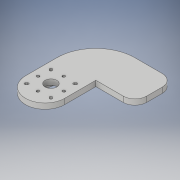
# Autodesk Inventor part: Motor Test Stand
Saved by Autodesk Inventor 2019 (Build 230136000, 136)
## iProperties
Created: 2019-09-23
Part Number: Motor Test Stand
Material: Generic
Document SubType Name: Modeling
Designer: isaac
Density: 1 g/cm^3
Appearance: Default
Author: isaac
Autodesk Inventor part; units mm, degrees
ref_plane "YZ Plane" through (0, 0, 0) normal (1, 0, 0) x (0, 1, 0)
ref_plane "XZ Plane" through (0, 0, 0) normal (0, 1, 0) x (-1, 0, 0)
ref_plane "XY Plane" through (0, 0, 0) normal (0, 0, 1) x (1, 0, 0)
sketch "Sketch1" plane through (0, 0, 0) normal (0, 1, 0) x (-1, 0, 0)
  line L0 (50, 65) -> (-50, 65)
  line L1 (-50, 65) -> (-50, -65)
  line L2 (-50, -65) -> (50, -65)
  line L3 (50, -65) -> (50, 65)
  line L4 (50, 65) -> (-50, -65) construction
  line L5 (-50, 65) -> (50, -65) construction
  point P0 (0, 0)
  dimension "d0" = 100
  dimension "d1" = 130
  constraints: 12 end point, 2 midpoint, 2 parallel, 1 horizontal, 1 perpendicular
  measures "d0" distance of L2.end L1.end
  measures "d1" distance of L1.end L0.end
extrude "Extrusion1" add sketch "Sketch1" along normal blind 7
sketch "Sketch2" plane through (0, 7, 0) normal (0, 1, 0) x (1, 0, 0)
  line L0 (-50, -65) -> (50, -65) projected
  line L1 (50, -65) -> (0, -65)
  line L2 (0, -65) -> (0, 0)
  line L3 (0, 0) -> (50, 0)
  line L4 (50, 0) -> (50, -65)
  constraints: 8 end point, 2 parallel, 1 horizontal, 1 perpendicular
extrude "Extrusion2" cut sketch "Sketch2" against normal up to next
fillet "Fillet1" radius 25 2 edges at (-50, 3.5, 65) (0, 3.5, 65)
sketch "Sketch5" plane through (0, 7, 0) normal (0, 1, 0) x (1, 0, 0)
  line L0 (-50, 65) -> (-50, -40) projected
  arc A0 (0, 50) -> (-50, 0) centre (0, 0) ccw
  line L1 (0, 50) -> (50, 50)
  line L2 (50, 0) -> (50, 65) projected
  line L3 (50, 50) -> (50, 65)
  line L4 (50, 65) -> (-50, 65) projected
  line L5 (50, 65) -> (-50, 65)
  line L6 (-50, 65) -> (-50, 0)
  constraints: 8 end point, 2 collinear, 2 point on circle, 1 centre point, 1 coincident, 1 horizontal, 1 perpendicular, 1 point on line, 1 tangent
extrude "Extrusion3" cut sketch "Sketch5" against normal up to next
fillet "Fillet2" radius 15 2 edges at (50, 3.5, 0) (50, 3.5, -50)
sketch "Sketch6" plane through (0, 7, 0) normal (0, 1, 0) x (1, 0, 0)
  arc A0 (0, 50) -> (-50, 0) centre (0, 0) ccw construction
  line L0 (-50, 0) -> (-25, -65) construction
  arc A1 (-50, -40) -> (0, -40) centre (-25, -40) ccw construction
  line L1 (0, -40) -> (0, 0) construction
  line L2 (0, 0) -> (-25, -65) construction
  line L3 (-25, -65) -> (-50, -65) construction
  line L4 (-50, 0) -> (-50, -40) construction
  line L5 (-50, -65) -> (-50, 0) construction
  line L6 (-25, -65) -> (0, -65) construction
  line L7 (0, -65) -> (0, 0) construction
  circle A2 centre (-25, -32.5) radius 22 construction
  line L8 (-47, -54.5) -> (-3, -54.5) construction
  line L9 (-3, -54.5) -> (-3, -10.5) construction
  line L10 (-3, -10.5) -> (-47, -10.5) construction
  line L11 (-47, -10.5) -> (-47, -54.5) construction
  line L12 (-47, -54.5) -> (-3, -10.5) construction
  line L13 (-3, -54.5) -> (-47, -10.5) construction
  line L14 (-41.0867, -48.5867) -> (-40.026, -47.526) construction
  line L15 (-39.973, -49.7004) -> (-38.9123, -48.6397)
  line L16 (-41.1397, -46.4123) -> (-42.2004, -47.473)
  arc A3 (-42.2004, -47.473) -> (-39.973, -49.7004) centre (-41.0867, -48.5867) ccw
  arc A4 (-38.9123, -48.6397) -> (-41.1397, -46.4123) centre (-40.026, -47.526) ccw
  line L17 (-41.0867, -16.4133) -> (-40.026, -17.474) construction
  line L18 (-42.2004, -17.527) -> (-41.1397, -18.5877)
  line L19 (-38.9123, -16.3603) -> (-39.973, -15.2996)
  arc A5 (-39.973, -15.2996) -> (-42.2004, -17.527) centre (-41.0867, -16.4133) ccw
  arc A6 (-41.1397, -18.5877) -> (-38.9123, -16.3603) centre (-40.026, -17.474) ccw
  line L20 (-8.9133, -48.5867) -> (-9.974, -47.526) construction
  line L21 (-7.7996, -47.473) -> (-8.8603, -46.4123)
  line L22 (-11.0877, -48.6397) -> (-10.027, -49.7004)
  arc A7 (-10.027, -49.7004) -> (-7.7996, -47.473) centre (-8.9133, -48.5867) ccw
  arc A8 (-8.8603, -46.4123) -> (-11.0877, -48.6397) centre (-9.974, -47.526) ccw
  line L23 (-8.9133, -16.4133) -> (-9.974, -17.474) construction
  line L24 (-10.027, -15.2996) -> (-11.0877, -16.3603)
  line L25 (-8.8603, -18.5877) -> (-7.7996, -17.527)
  arc A9 (-7.7996, -17.527) -> (-10.027, -15.2996) centre (-8.9133, -16.4133) ccw
  arc A10 (-11.0877, -16.3603) -> (-8.8603, -18.5877) centre (-9.974, -17.474) ccw
  circle A11 centre (-25, -32.5) radius 16.5 construction
  line L26 (-47, -32.5) -> (-3, -32.5) construction
  line L27 (-25, -54.5) -> (-25, -10.5) construction
  line L28 (-41.75, -32.5) -> (-41.25, -32.5) construction
  line L29 (-41.75, -34.075) -> (-41.25, -34.075)
  line L30 (-41.25, -30.925) -> (-41.75, -30.925)
  arc A12 (-41.75, -30.925) -> (-41.75, -34.075) centre (-41.75, -32.5) ccw
  arc A13 (-41.25, -34.075) -> (-41.25, -30.925) centre (-41.25, -32.5) ccw
  line L31 (-25, -49.25) -> (-25, -48.75) construction
  line L32 (-23.425, -49.25) -> (-23.425, -48.75)
  line L33 (-26.575, -48.75) -> (-26.575, -49.25)
  arc A14 (-26.575, -49.25) -> (-23.425, -49.25) centre (-25, -49.25) ccw
  arc A15 (-23.425, -48.75) -> (-26.575, -48.75) centre (-25, -48.75) ccw
  line L34 (-8.25, -32.5) -> (-8.75, -32.5) construction
  line L35 (-8.25, -30.925) -> (-8.75, -30.925)
  line L36 (-8.75, -34.075) -> (-8.25, -34.075)
  arc A16 (-8.25, -34.075) -> (-8.25, -30.925) centre (-8.25, -32.5) ccw
  arc A17 (-8.75, -30.925) -> (-8.75, -34.075) centre (-8.75, -32.5) ccw
  line L37 (-25, -15.75) -> (-25, -16.25) construction
  line L38 (-26.575, -15.75) -> (-26.575, -16.25)
  line L39 (-23.425, -16.25) -> (-23.425, -15.75)
  arc A18 (-23.425, -15.75) -> (-26.575, -15.75) centre (-25, -15.75) ccw
  arc A19 (-26.575, -16.25) -> (-23.425, -16.25) centre (-25, -16.25) ccw
  circle A20 centre (-25, -32.5) radius 7.5
  point P0 (-40.5563, -48.0563)
  point P1 (-40.5563, -16.9437)
  point P2 (-9.4437, -48.0563)
  point P3 (-9.4437, -16.9437)
  point P4 (-41.5, -32.5)
  point P5 (-25, -49)
  point P6 (-8.5, -32.5)
  point P7 (-25, -16)
  dimension "d18" = 44
  dimension "d19" = 44
  dimension "d20" = 44
  dimension "d21" = 0.75
  dimension "d22" = 3.15
  dimension "d23" = 0.75
  dimension "d24" = 3.15
  dimension "d25" = 0.75
  dimension "d26" = 3.15
  dimension "d27" = 0.75
  dimension "d28" = 3.15
  dimension "d29" = 33
  dimension "d30" = 0.25
  dimension "d31" = 3.15
  dimension "d32" = 0.25
  dimension "d33" = 3.15
  dimension "d34" = 0.25
  dimension "d35" = 3.15
  dimension "d36" = 0.25
  dimension "d37" = 3.15
  dimension "d38" = 15
  constraints: 92 end point, 41 point on circle, 33 tangent, 19 centre point, 16 point on line, 14 midpoint, 10 parallel, 3 horizontal, 2 coincident, 2 perpendicular, 1 collinear
  measures "d18" diameter of A2
  measures "d19" distance of L10.end L9.end
  measures "d20" distance of L9.end L8.end
  measures "d21" distance of A2.start L14.end
  measures "d22" diameter of A4
  measures "d23" distance of A2.end L17.end
  measures "d24" diameter of A6
  measures "d25" distance of point (-9.444, -48.056) L20.end
  measures "d26" diameter of A8
  measures "d27" distance of point (-9.444, -16.944) L23.end
  measures "d28" diameter of A10
  measures "d29" diameter of A11
  measures "d30" distance of A11.start L28.end
  measures "d31" diameter of A13
  measures "d32" distance of A11.end L31.end
  measures "d33" diameter of A15
  measures "d34" distance of point (-8.5, -32.5) L34.end
  measures "d35" diameter of A17
  measures "d36" distance of point (-25, -16) L37.end
  measures "d37" diameter of A19
  measures "d38" diameter of A20
extrude "Extrusion4" cut sketch "Sketch6" against normal up to next
sketch "Sketch7" plane through (0, 0, 0) normal (0, -1, 0) x (1, 0, 0)
  line L0 (-11.5874, 0) -> (-11.5874, 58.918) construction
  line L1 (-11.5874, 58.918) -> (-17.5, 58.918) construction
  line L2 (-17.5, 58.918) -> (-17.5, 0) construction
  line L3 (-16.4027, 0) -> (-12.8001, 0)
  line L4 (-12.8001, 0) -> (-12.8001, 55)
  line L5 (-12.8001, 55) -> (-16.4027, 55)
  line L6 (-16.4027, 55) -> (-16.4027, 0)
  circle A0 centre (-25, 32.5) radius 7.5 construction
  line L7 (-25, 32.5) -> (-25, 62.0042) construction
  line L8 (-33.5973, 0) -> (-37.1999, 0)
  line L9 (-37.1999, 55) -> (-33.5973, 55)
  line L10 (-33.5973, 55) -> (-33.5973, 0)
  line L11 (-37.1999, 0) -> (-37.1999, 55)
  point P0 (0, 0)
  dimension "d41" = 55
  constraints: 24 end point, 4 symmetric about line, 3 parallel, 1 perpendicular, 1 vertical
  measures "d41" distance of L4.end L3.end
extrude "Extrusion5" add sketch "Sketch7" along normal blind 7
sketch "Sketch8" plane through (-12.8001, 0, 55) normal (1, 0, 0) x (0, 0, -1)
  line L0 (55, -7) -> (0, -7) projected
  line L1 (0, 0) -> (0, -7) projected
  line L2 (45, -7) -> (0, 0)
  line L3 (0, 0) -> (0, -7)
  line L4 (0, -7) -> (45, -7)
  point P0 (55, 0)
  constraints: 6 end point, 1 perpendicular, 1 point on line, 1 vertical
extrude "Extrusion6" cut sketch "Sketch8" against normal through all
body "Solid1"
